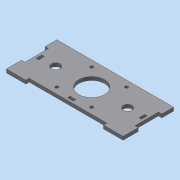
# Autodesk Inventor part: X-Motor-Housing_Front-Inner
Saved by Autodesk Inventor 2016 SP1 (Build 200210100, 210)
## iProperties
Created: 2015-12-01
Part Number: X-Motor-Housing_Front-Inner
Material: Generic
Document SubType Name: Modeling
Designer: Mohamed A.
Density: 1 g/cm^3
Appearance: Default
Mass: 9.73173 g
Surface Area: 83.8715 cm^2
Volume: 9.73173 cm^3
Author: Mohamed A.
Autodesk Inventor part; units mm, degrees
ref_plane "YZ Plane" through (0, 0, 0) normal (1, 0, 0) x (0, 1, 0)
ref_plane "XZ Plane" through (0, 0, 0) normal (0, 1, 0) x (-1, 0, 0)
ref_plane "XY Plane" through (0, 0, 0) normal (0, 0, 1) x (1, 0, 0)
sketch "Sketch1" plane through (0, 0, 0) normal (0, 0, 1) x (1, 0, 0)
  line L0 (49, 21) -> (-49, 21)
  line L1 (-49, -21) -> (-21, -21)
  circle A0 centre (32, 0) radius 3.9
  circle A1 centre (-32, 0) radius 3.9
  line L2 (49, 21) -> (49, 10.5)
  line L3 (-49, -21) -> (-49, -10.5)
  line L4 (0, 41.7106) -> (0, -39.2634) construction
  line L5 (-50.5476, 0) -> (60.8869, 0) construction
  circle A2 centre (0, 0) radius 11.5
  line L6 (21, 21) -> (21, -21) construction
  line L7 (-21, -21) -> (-21, 21) construction
  line L8 (49, 21) -> (52, 21)
  line L9 (52, 21) -> (52, 10.5)
  line L10 (52, -21) -> (49, -21)
  line L11 (49, 10.5) -> (52, 10.5)
  line L12 (49, -10.5) -> (52, -10.5)
  line L13 (49, 10.5) -> (49, -10.5)
  line L14 (49, -10.5) -> (49, -21)
  line L15 (52, -10.5) -> (52, -21)
  line L16 (52, 10.5) -> (52, -10.5)
  line L17 (44.6, 2.65) -> (47, 2.65)
  line L18 (47, 2.65) -> (47, -2.65)
  line L19 (47, -2.65) -> (44.6, -2.65)
  line L20 (44.6, -2.65) -> (44.6, 2.65)
  line L21 (-49, 21) -> (-52, 21)
  line L22 (-52, 21) -> (-52, 10.5)
  line L23 (-49, 10.5) -> (-52, 10.5)
  line L24 (-49, -10.5) -> (-52, -10.5)
  line L25 (-52, -10.5) -> (-52, -21)
  line L26 (-52, 10.5) -> (-52, -10.5)
  line L27 (-44.6, 2.65) -> (-47, 2.65)
  line L28 (-47, 2.65) -> (-47, -2.65)
  line L29 (-47, -2.65) -> (-44.6, -2.65)
  line L30 (-44.6, -2.65) -> (-44.6, 2.65)
  line L31 (-52, -21) -> (-49, -21)
  line L32 (-49, 10.5) -> (-49, 21)
  line L33 (-49, -10.5) -> (-49, 10.5)
  line L34 (52, -21) -> (52, -24)
  line L35 (52, -24) -> (-52, -24)
  line L36 (-52, -24) -> (-52, -21)
  line L37 (34.6667, -24) -> (34.6667, -21)
  line L38 (-34.6667, -24) -> (-34.6667, -21)
  line L39 (-2.65, -16.6) -> (2.65, -16.6)
  line L40 (2.65, -16.6) -> (2.65, -19)
  line L41 (2.65, -19) -> (-2.65, -19)
  line L42 (-2.65, -19) -> (-2.65, -16.6)
  line L43 (21, -21) -> (49, -21)
  line L44 (-21, -21) -> (21, -21)
  circle A3 centre (-15.5, 15.5) radius 1.4
  circle A4 centre (-15.5, -15.5) radius 1.4
  circle A5 centre (15.5, -15.5) radius 1.4
  circle A6 centre (15.5, 15.5) radius 1.4
  dimension "d4" = 7.8
  dimension "d5" = 7.8
  dimension "d111" = 42
  dimension "d115" = 21
  dimension "d116" = 21
  dimension "d117" = 23
  dimension "d118" = 42
  dimension "d123" = 3
  dimension "d124" = 21
  dimension "d125" = 5.3
  dimension "d126" = 2.4
  dimension "d128" = 5
  dimension "d129" = 3
  dimension "d130" = 104
  dimension "d131" = 69.3333
  dimension "d132" = 5.3
  dimension "d133" = 2.4
  dimension "d134" = 5
  dimension "d135" = 2.8
  dimension "d136" = 5.5
  dimension "d137" = 5.5
  dimension "d140" = 360
  dimension "d143" = 12.6
  constraints: 90 end point, 26 perpendicular, 10 point on line, 10 symmetric about line, 7 centre point, 6 vertical, 4 horizontal, 4 parallel, 1 coincident, 16 other
  measures "d4" diameter of A0
  measures "d5" diameter of A1
  measures "d111" distance between parallel lines of L1 L0
  measures "d115" distance from line of A0.centre L0
  measures "d116" distance from line of A1.centre L0
  measures "d117" diameter of A2
  measures "d118" distance between parallel lines of L7 L6
  measures "d123" distance between parallel lines of L2 L9
  measures "d124" distance between parallel lines of L12 L11
  measures "d125" distance between parallel lines of L19 L17
  measures "d126" distance between parallel lines of L20 L18
  measures "d128" distance between parallel lines of L16 L18
  measures "d129" distance of L10.start L34.end
  measures "d130" distance between parallel lines of L36 L34
  measures "d131" distance between parallel lines of L38 L37
  measures "d132" distance of L40.end L41.end
  measures "d133" distance of L39.end L40.end
  measures "d134" distance between parallel lines of L35 L41
  measures "d135" diameter of A3
  measures "d136" distance from line of L0 A3.centre
  measures "d137" distance from line of L7 A3.centre
  measures "d143" distance from line of A0.centre L20
extrude "Extrusion1" add sketch "Sketch1" against normal blind 3 contours L2 L13 L14 L43 L44 L1 L3 L33 L32 L0 | L8 L9 L11 L2 | L32 L23 L22 L21 | L12 L15 L10 L14 | L3 L31 L25 L24 | L10 L34 L35 L37 L43 | L1 L38 L35 L36 L31
body "Solid1"
